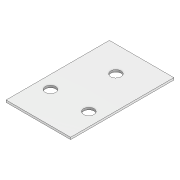
# Autodesk Inventor part: 2020-04-02-10-10401-Outline_ConnectorPCB
Saved by Autodesk Inventor 2020 (Build 240168000, 168)
## iProperties
Created: 2020-11-03
Part Number: 2020-04-02-10-10401-Outline_ConnectorPCB
Material: ABS Plastic
Document SubType Name: Modeling
Designer: eunde
Density: 1.06 g/cm^3
Appearance: Smooth - White
Author: eunde
Autodesk Inventor part; units mm, degrees
ref_plane "YZ Plane" through (0, 0, 0) normal (1, 0, 0) x (0, 1, 0)
ref_plane "XZ Plane" through (0, 0, 0) normal (0, 1, 0) x (-1, 0, 0)
ref_plane "XY Plane" through (0, 0, 0) normal (0, 0, 1) x (1, 0, 0)
sketch "Sketch1" plane through (0, 0, 0) normal (0, 1, 0) x (-1, 0, 0)
  line L0 (0, 0) -> (-50, 0)
  line L1 (-50, 0) -> (-50, 80)
  line L2 (-50, 80) -> (0, 80)
  line L3 (0, 80) -> (0, 0)
  dimension "d0" = 50
  dimension "d1" = 80
  constraints: 8 end point, 2 parallel, 1 horizontal, 1 perpendicular
  measures "d0" distance of L1.end L2.end
  measures "d1" distance of L0.end L1.end
extrude "Extrusion1" add sketch "Sketch1" along normal blind 1.6
sketch "Sketch2" plane through (0, 1.6, 0) normal (0, 1, 0) x (1, 0, 0)
  circle A0 centre (10.152, -55.746) radius 4
  line L0 (0, 0) -> (0, -80) projected
  line L1 (50, 0) -> (0, 0) projected
  line L2 (0, -80) -> (50, -80) projected
  circle A1 centre (39.85, -55.746) radius 4
  circle A2 centre (25, -19.9) radius 4
  point P0 (25, -80)
  dimension "d4" = 10.152
  dimension "d5" = 8
  dimension "d9" = 24.254
  dimension "d10" = 8
  dimension "d11" = 29.698
  dimension "d12" = 8
  dimension "d13" = 19.9
  constraints: 3 centre point, 1 horizontal alignment, 1 midpoint, 1 vertical alignment
  measures "d4" distance from line of L0 A0.centre
  measures "d5" diameter of A0
  measures "d9" distance from line of L2 A0.centre
  measures "d10" diameter of A1
  measures "d11" distance of A0.centre A1.centre
  measures "d12" diameter of A2
  measures "d13" distance from line of L1 A2.centre
extrude "Holes for" cut sketch "Sketch2" against normal blind 10
equation "\"d12\" = d10"
body "Solid1"
